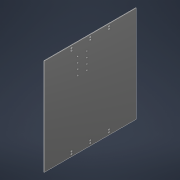
# Autodesk Inventor part: BottomV4
Saved by Autodesk Inventor 2022 (Build 260153000, 153)
## iProperties
Created: 2021-10-02
Part Number: BottomV4
Material: Steel
Document SubType Name: Sheet Metal
Designer: timmy
Density: 7.85 g/cm^3
Appearance: Smooth - Black
Sheet Metal Rule: Default
Author: timmy
Autodesk Inventor part; units mm, degrees
ref_plane "YZ Plane" through (0, 0, 0) normal (1, 0, 0) x (0, 1, 0)
ref_plane "XZ Plane" through (0, 0, 0) normal (0, 1, 0) x (-1, 0, 0)
ref_plane "XY Plane" through (0, 0, 0) normal (0, 0, 1) x (1, 0, 0)
sketch "Sketch1" plane through (0, 0, 0) normal (1, 0, 0) x (0, 1, 0)
  line L0 (0, 0) -> (533.4, 0)
  line L1 (533.4, 0) -> (533.4, -508)
  line L2 (533.4, -508) -> (0, -508)
  line L3 (0, -508) -> (0, 0)
  dimension "d0" = 533.4
  dimension "d1" = 508
  constraints: 8 end point, 2 parallel, 1 horizontal, 1 perpendicular
  measures "d0" distance of L1.end L2.end
  measures "d1" distance of L0.end L1.end
extrude "Extrusion1" add sketch "Sketch1" along normal blind 1.5875
sketch "Sketch3" plane through (0, 0, 0) normal (-1, 0, 0) x (0, 0, 1)
  line L0 (-508, 0) -> (-508, 533.4) projected
  line L1 (0, 0) -> (-508, 0) projected
  circle A0 centre (-358.14, 12.7) radius 3.302
  circle A1 centre (-358.14, 25.4) radius 3.302
  circle A2 centre (-149.86, 12.7) radius 3.302
  circle A3 centre (-149.86, 25.4) radius 3.302
  circle A4 centre (-254, 12.7) radius 3.302
  circle A5 centre (-254, 25.4) radius 3.302
  circle A6 centre (-358.14, 508) radius 3.302
  circle A7 centre (-358.14, 520.7) radius 3.302
  circle A8 centre (-149.86, 508) radius 3.302
  circle A9 centre (-149.86, 520.7) radius 3.302
  circle A10 centre (-254, 508) radius 3.302
  circle A11 centre (-254, 520.7) radius 3.302
  constraints: 12 centre point
extrude "Extrusion5" cut sketch "Sketch3" against normal up to surface (1.5875 mm away) contours A0 | A1 | A2 | A3 | A4 | A5
sheet face with bend "Face1" sketch "Sketch1" thickness 3.048 toward (1, 0, 0) bend radius 3.048
bend "Bend1"
extrude "Cut1" cut sketch "Sketch3" against normal up to surface (3.048 mm away)
sketch "Sketch4" plane through (0, 0, 0) normal (-1, 0, 0) x (0, 0, 1)
  circle A0 centre (-184.0615, 463.1989) radius 2.3495
  line L0 (-184.0615, 463.1989) -> (-234.8615, 463.1989)
  circle A1 centre (-234.8615, 463.1989) radius 2.3495
  line L1 (-184.0615, 463.1989) -> (-184.0615, 447.9589)
  line L2 (-184.0615, 447.9589) -> (-184.0615, 432.7189)
  circle A2 centre (-184.0615, 432.7189) radius 2.3495
  circle A3 centre (-234.8615, 432.7189) radius 2.3495
  line L3 (-184.0615, 432.7189) -> (-184.0615, 417.4789)
  line L4 (-184.0615, 417.4789) -> (-184.0615, 402.2389)
  line L5 (-184.0615, 402.2389) -> (-234.8615, 402.2389)
  line L6 (-234.8615, 402.2389) -> (-234.8615, 386.9989)
  line L7 (-234.8615, 386.9989) -> (-234.8615, 371.7589)
  line L8 (-234.8615, 371.7589) -> (-184.0615, 371.7589)
  circle A4 centre (-184.0615, 402.2389) radius 2.3495
  circle A5 centre (-234.8615, 402.2389) radius 2.3495
  circle A6 centre (-234.8615, 371.7589) radius 2.3495
  circle A7 centre (-184.0615, 371.7589) radius 2.3495
  point P0 (0, 0)
  dimension "d47" = 50.8
  dimension "d48" = 4.699
  dimension "d49" = 15.24
  dimension "d50" = 15.24
  dimension "d51" = 4.699
  dimension "d52" = 4.699
  dimension "d53" = 15.24
  dimension "d54" = 15.24
  dimension "d55" = 15.24
  dimension "d56" = 15.24
  dimension "d57" = 4.699
  dimension "d58" = 4.699
  dimension "d59" = 4.699
  dimension "d60" = 4.699
  constraints: 18 end point, 8 centre point, 6 coincident, 4 point on line, 3 perpendicular, 2 vertical, 1 horizontal
  measures "d47" distance of L0.start L0.end
  measures "d48" diameter of A1
  measures "d49" distance of L0.start L1.end
  measures "d50" distance of L1.end L2.end
  measures "d51" diameter of A2
  measures "d52" diameter of A3
  measures "d53" distance of L3.start L3.end
  measures "d54" distance of L3.end L4.end
  measures "d55" distance of L5.end L6.end
  measures "d56" distance of L6.end L7.end
  measures "d57" diameter of A4
  measures "d58" diameter of A5
  measures "d59" diameter of A6
  measures "d60" diameter of A7
extrude "Cut2" cut sketch "Sketch4" against normal blind 3.048
equation "\"d38\" = Thickness"
equation "\"d43\" = Thickness"
equation "\"d32\" = Thickness"
equation "\"d33\" = BendRadius"
equation "\"d34\" = BendReliefWidth"
equation "\"d36\" = MinimumRemnant"
equation "\"d35\" = BendReliefDepth"
equation "\"d37\" = TransitionRadius"
equation "\"BendRadius\" = Thickness"
equation "\"BendReliefWidth\" = Thickness"
equation "\"BendReliefDepth\" = 0.5 * Thickness"
equation "\"CornerReliefSize\" = 4 * Thickness"
equation "\"MinimumRemnant\" = 2 * Thickness"
equation "\"TransitionRadius\" = BendRadius"
equation "\"JacobiRadiusSize\" = BendRadius"
equation "\"GapSize\" = Thickness"
equation "\"Thickness\" = 3.048"
body "Solid1"
